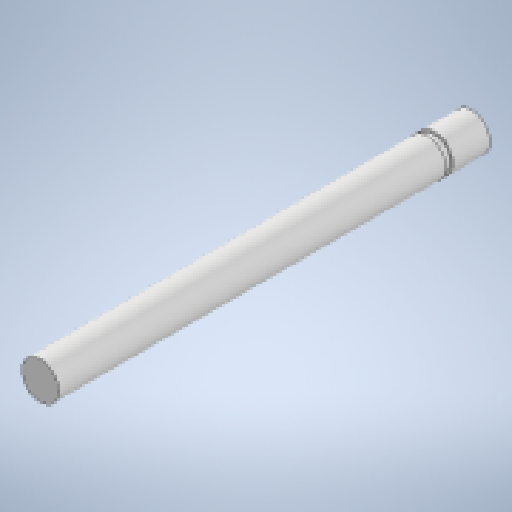
# Autodesk Inventor part: wał_2
Saved by Autodesk Inventor 2023 (Build 270158000, 158)
## iProperties
Created: 2023-03-11
Part Number: wał_2
Material: Ogólny
Document SubType Name: Modeling
Designer: Kamil
Density: 1 g/cm^3
Appearance: Domyślna
Author: Kamil
Autodesk Inventor part; units mm, degrees
ref_plane "YZ Plane" through (0, 0, 0) normal (1, 0, 0) x (0, 1, 0)
sketch "Szkic1" plane through (0, 0, 0) normal (0, 0, 1) x (1, 0, 0)
  circle A0 centre (-2.912, -2.7423) radius 5.3 projected
  circle A1 centre (-2.912, -2.7423) radius 5
  point P0 (0, 0)
  dimension "d0" = 10
  constraints: 1 centre point, 1 coincident
  measures "d0" diameter of A1
extrude "Wyciągnięcie proste1" add sketch "Szkic1" along normal blind 120 contours A1
sketch "Szkic2" plane through (-2.912, -2.7423, 5) normal (0, 0, -1) x (-1, 0, 0)
  circle A0 centre (0, 0) radius 5 projected
  circle A1 centre (0, 0) radius 4.284
  point P0 (-2.912, 2.7423)
  constraints: 1 centre point, 1 coincident
ref_plane "Płaszczyzna konstrukcyjna1" through (-12.2191, -12.0493, 11.96) normal (0, 0, -1) x (-0.4239, 0.9057, 0)
extrude "Wyciągnięcie proste2" cut sketch "Szkic2" against normal up to surface (6.96 mm away)
extrude "Wyciągnięcie proste3" cut sketch "Szkic2" against normal blind 5 contours A1
sketch "Szkic3" plane through (-2.912, -2.7423, 10) normal (0, 0, -1) x (-1, 0, 0)
  circle A0 centre (0, 0) radius 4.284 projected
  circle A1 centre (0, 0) radius 4.284 projected
  circle A2 centre (0, 0) radius 5 projected
  point P0 (-2.912, 2.7423)
ref_plane "Płaszczyzna konstrukcyjna2" through (-9.0993, -8.9295, 0) normal (0, 0, 1) x (1, 0, 0)
extrude "Wyciągnięcie proste4" add sketch "Szkic3" along normal up to surface (10 mm away) contours A0 | A2
sketch "Szkic4" plane through (-2.912, -2.7423, 11.96) normal (0, 0, -1) x (-1, 0, 0)
  circle A0 centre (0, 0) radius 5 projected
  circle A1 centre (0, 0) radius 6
  point P0 (-2.912, 2.7423)
  dimension "d15" = 12
  constraints: 1 centre point, 1 coincident
  measures "d15" diameter of A1
extrude "Wyciągnięcie proste5" add sketch "Szkic4" along normal blind 2 contours A0 | A1
sketch "Szkic5" plane through (-2.912, -2.7423, 9.96) normal (0, 0, -1) x (-1, 0, 0)
  circle A0 centre (0, 0) radius 5 projected
  circle A1 centre (0, 0) radius 5 projected
  circle A2 centre (0, 0) radius 5
  point P0 (-2.912, 2.7423)
  constraints: 1 centre point, 1 coincident, 1 concentric
extrude "Wyciągnięcie proste6" add sketch "Szkic5" along normal blind 25
sketch "Szkic6" plane through (-2.912, -2.7423, 116) normal (0, 0, 1) x (1, 0, 0)
  circle A0 centre (0, 0) radius 5 projected
  point P0 (2.912, 2.7423)
extrude "Wyciągnięcie proste7" add sketch "Szkic6" along normal blind 15
sketch "Szkic7" plane through (-2.912, -2.7423, 131) normal (0, 0, 1) x (1, 0, 0)
  circle A0 centre (0, 0) radius 5 projected
  point P0 (2.912, 2.7423)
extrude "Wyciągnięcie proste8" cut sketch "Szkic7" against normal blind 0.04
